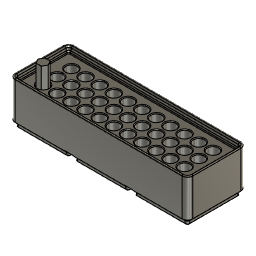
Bit holder v4 (Autodesk Fusion 360 design; units mm, degrees)
Autodesk Fusion 360 part; units mm, degrees
note: some values were not read from the file. Set by a fixed rule: which face or edge a step refers to.
sketch "Sketch1" plane through (0, 0, 0) normal (0, 0, 1) x (1, 0, 0) in component "Standard Bit"
  line L0 (-1.8331, 3.175) -> (-3.6662, 0)
  line L1 (-3.6662, 0) -> (-1.8331, -3.175)
  line L2 (-1.8331, -3.175) -> (1.8331, -3.175)
  line L3 (1.8331, -3.175) -> (3.6662, 0)
  line L4 (3.6662, 0) -> (1.8331, 3.175)
  line L5 (1.8331, 3.175) -> (-1.8331, 3.175)
  dimension "d234" = 6.35
  measures "d234" distance of L2 L5
extrude "Extrude2" add sketch "Sketch1" along normal blind 8 makes body 1 in component "Standard Bit"
chamfer "Chamfer1" distance 1 angle 45 6 edges at (-2.7496, -1.5875, 0) (0, -3.175, 0) (2.7496, -1.5875, 0) (2.7496, 1.5875, 0) (0, 3.175, 0) (-2.7496, 1.5875, 0) on bodies 1 in component "Standard Bit"
sketch "Sketch2" plane through (0, 0, 8) normal (0, 0, 1) x (-1, 0, 0) in component "Standard Bit"
  line L0 (-1.8331, -3.175) -> (1.8331, -3.175)
  line L1 (1.8331, -3.175) -> (3.6662, 0)
  line L2 (3.6662, 0) -> (1.8331, 3.175)
  line L3 (1.8331, 3.175) -> (-1.8331, 3.175)
  line L4 (-1.8331, 3.175) -> (-3.6662, 0)
  line L5 (-3.6662, 0) -> (-1.8331, -3.175)
  circle A0 centre (0, 0) radius 3.6662
  constraint coincident A0.centre origin
  constraint coincident L0.start A0
extrude "Extrude1" add sketch "Sketch1" along normal blind 17 from surface at 8 bodies 1 in component "Standard Bit"
pipe "Pipe1" cut square section size 0.5 path "Sketch2" along A0 bodies 1 in component "Standard Bit"
sketch "Sketch1 (2)" plane through (0, 0, 0) normal (0, 0, 1) x (1, 0, 0) in component "Blank Storage"
  line L0 (0, 42) -> (42, 42)
  line L1 (42, 42) -> (42, 0)
  line L2 (42, 0) -> (0, 0)
  line L3 (0, 0) -> (0, 42)
  line L4 (0, 42) -> (42, 0) construction
  line L5 (42, 21) -> (0, 21) construction
  line L6 (42, 14.5) -> (0, 14.5)
  line L7 (42, 27.5) -> (0, 27.5)
  line L8 (27.5, 42) -> (27.5, 0)
  line L9 (14.5, 42) -> (14.5, 0)
  line L10 (14.5, 14.5) -> (0, 0) construction
  circle A0 centre (8, 8) radius 1.5
  circle A1 centre (34, 8) radius 1.5
  circle A2 centre (34, 34) radius 1.5
  circle A3 centre (8, 34) radius 1.5
  circle A4 centre (8, 8) radius 3.25
  circle A5 centre (34, 8) radius 3.25
  circle A6 centre (34, 34) radius 3.25
  circle A7 centre (8, 34) radius 3.25
  line L11 (6.5, 10.8831) -> (6.5, 5.1169)
  line L12 (5.1169, 6.5) -> (10.8831, 6.5)
  line L13 (9.5, 5.1169) -> (9.5, 10.8831)
  line L14 (10.8831, 9.5) -> (5.1169, 9.5)
  point P0 (21, 21)
  dimension "d1" = 42
  dimension "d2" = 42
  dimension "d65" = 13
  dimension "d67" = 90
  dimension "d69" = 3
  dimension "d71" = 360
  dimension "d80" = 6.5
  dimension "d85" = 8
  constraint horizontal L0
  constraint perpendicular L0 L1
  constraint parallel L0 L2
  constraint parallel L1 L3
  constraint coincident L2.end L3.start
  constraint midpoint L1 L5.start
  constraint midpoint L3 L5.end
  constraint coincident L1 L6.start
  constraint coincident L3 L6.end
  constraint perpendicular L3 L6
  constraint symmetric L5 L6.start L7.start
  constraint symmetric L5 L6.end L7.end
  constraint midpoint L4 P0
  constraint coincident L9 L10.start
  constraint coincident L6 L10.start
  constraint concentric A0 A4
  constraint coincident L10 A0.centre
  constraint coincident A4 L11.start
  constraint coincident A4 L11.end
  constraint coincident A4 L12.start
  constraint coincident A4 L12.end
  constraint coincident A4 L13.start
  constraint coincident A4 L13.end
  constraint coincident A4 L14.start
  constraint coincident A4 L14.end
  constraint horizontal L12
  constraint horizontal L14
  constraint vertical L13
  constraint vertical L11
  constraint tangent A0 L11
  constraint tangent A0 L12
  constraint tangent A0 L13
  constraint tangent A0 L14
  measures "d1" distance of L1.end L2.end
  measures "d2" distance of L0.end L1.end
  measures "d65" distance of L6 L7
  measures "d69" diameter of A0
  measures "d80" diameter of A4
  measures "d85" distance of L2 A0.centre
extrude "Extrude1'" add sketch "Sketch1 (2)" along normal blind 5 separate body contours L0 L3 L7 L9 | L0 L7 L8 L9 | L3 L6 L7 L9 | L0 L1 L7 L8 | L6 L7 L8 L9 | L2 L3 L6 L9 | L1 L6 L7 L8 | L2 L6 L8 L9 | L1 L2 L6 L8 | A0 | A0 L12 L13 | A4 L12 L13 L14 | A0 L13 L14 | A4 L11 L13 L14 | A0 L11 L14 | A0 L11 L12 | A4 L11 L12 L13 | A4 L12 L13 | A4 L13 L14 | A4 L11 L12 L14 | A4 L11 L14 | A4 L11 L12 | A1 | A2 | A3 | A5 | A6 | A7 makes body 2 in component "Blank Storage"
ref_plane "WorkPlane1" through (21, 21, 2.5) normal (0, -1, 0) x (1, 0, 0) in component "Blank Storage"
sketch "Sketch2 (2)" plane through (0, 21, 0) normal (0, -1, 0) x (1, 0, 0) in component "Blank Storage"
  line L0 (42, 0) -> (0, 0)
  line L1 (0, 0) -> (0, 5)
  line L2 (3.2, 0) -> (2.4, 0.8)
  line L3 (3.2, 0) -> (0, 0) construction
  line L4 (2.4, 0.8) -> (2.4, 2.6)
  line L5 (2.4, 2.6) -> (0, 5)
  line L6 (0, 5) -> (-5.1222, 5)
  line L7 (-5.1222, 5) -> (-5.1222, -0.0937)
  line L8 (-5.1222, -0.0937) -> (0, 0)
  dimension "d39" = 45
  dimension "d40" = 45
  dimension "d41" = 0.8
  dimension "d43" = 5
  dimension "d112" = 2.4
  constraint horizontal L3
  constraint coincident L0 L2.start
  constraint perpendicular L0 L4
  constraint coincident L1 L5.end
  constraint coincident L0.end L1.start
  constraint coincident L1.end L5.end
  constraint perpendicular L1 L6
  constraint perpendicular L6 L7
  measures "d39" angle of L2 L3
  measures "d40" angle of L4 L5
  measures "d41" distance of L2.end L3
  measures "d43" distance of L3 L1.end
  measures "d112" horizontal distance of L0.end L2.end
sketch "Sketch3" plane through (0, 0, 0) normal (0, 0, -1) x (1, 0, 0) in component "Storage Template v5"
  line L0 (42, 0) -> (0, 0)
  line L1 (0, 0) -> (0, -42)
  line L2 (0, -42) -> (42, -42)
  line L3 (42, -42) -> (42, 0)
  arc A0 (4, 0) -> (0, -4) centre (4, -4) ccw
  line L4 (0, -42) -> (42, 0) construction
  arc A1 (0, -38) -> (4, -42) centre (4, -38) ccw
  arc A2 (38, -42) -> (42, -38) centre (38, -38) ccw
  arc A3 (42, -4) -> (38, 0) centre (38, -4) ccw
  line L5 (0, -4) -> (0, -38)
  line L6 (4, -42) -> (38, -42)
  line L7 (42, -38) -> (42, -4)
  line L8 (38, 0) -> (4, 0)
  point P0 (21, -21)
  dimension "d37" = 360
  constraint coincident L1.end L2.start
  constraint coincident L0.start L3.end
  constraint midpoint L4 P0
sweep "Sweep1" cut profiles "Sketch2 (2)" path "Sketch3" along L8 A0 L5 A1 L6 A2 L7 A3 section 1 bodies 2 in component "Blank Storage"
extrude "Extrude3" [suppressed] in component "Blank Storage"
draft "Draft1" [suppressed] in component "Blank Storage"
extrude "Extrude4" cut sketch "Sketch1 (2)" along normal up to surface (5 mm away) contours A0 | A1 | A2 | A3 bodies 2 in component "Blank Storage"
extrude "Extrude5" cut sketch "Sketch1 (2)" along normal blind 2.4 contours A0 L12 L13 | A4 L12 L13 L14 | A0 L13 L14 | A4 L11 L13 L14 | A0 L11 L14 | A0 L11 L12 | A4 L11 L12 L13 | A4 L12 L13 | A4 L13 L14 | A4 L11 L12 L14 | A4 L11 L14 | A4 L11 L12 | A5 | A6 | A7 bodies 2 in component "Blank Storage"
extrude "Extrude8" cut sketch "Sketch1 (2)" along normal blind 0.25 from surface at 2.4 contours A0 L12 L13 | A4 L12 L13 L14 | A0 L13 L14 | A0 L11 L14 | A0 L11 L12 | A4 L11 L12 L14 bodies 2 in component "Blank Storage"
extrude "Extrude9" cut sketch "Sketch1 (2)" along normal blind 0.25 from surface at 2.65 contours A0 L12 L13 | A0 L13 L14 | A4 L11 L13 L14 | A0 L11 L14 | A0 L11 L12 | A4 L11 L12 L13 bodies 2 in component "Blank Storage"
pattern_circular "C-Pattern1" count 4 over 360 about axis through (21, 21, -42) along (0, 0, 1) of "Extrude8", "Extrude9" in component "Blank Storage"
pattern_linear "R-Pattern1" count 3 spacing 42 along (1, 0, 0) of bodies 2 makes body 3 at (66.9668, 17.0068, 5) makes body 4 at (108.9668, 17.0068, 5) in component "Blank Storage"
sketch "Sketch4" plane through (0, 0, 5) normal (0, 0, 1) x (-1, 0, 0) in component "Blank Storage"
  line L0 (-4, 0) -> (-122, 0)
  line L1 (-126, -4) -> (-126, -38)
  line L2 (-122, -42) -> (-4, -42)
  line L3 (0, -38) -> (0, -4)
  arc A0 (0, -4) -> (-4, 0) centre (-4, -4) ccw
  arc A1 (-122, 0) -> (-126, -4) centre (-122, -4) ccw
  arc A2 (-126, -38) -> (-122, -42) centre (-122, -38) ccw
  arc A3 (-4, -42) -> (0, -38) centre (-4, -38) ccw
  line L4 (-122, -41.75) -> (-4, -41.75)
  arc A4 (-4, -41.75) -> (-0.25, -38) centre (-4, -38) ccw
  line L5 (-0.25, -38) -> (-0.25, -4)
  arc A5 (-0.25, -4) -> (-4, -0.25) centre (-4, -4) ccw
  line L6 (-4, -0.25) -> (-122, -0.25)
  arc A6 (-122, -0.25) -> (-125.75, -4) centre (-122, -4) ccw
  line L7 (-125.75, -4) -> (-125.75, -38)
  arc A7 (-125.75, -38) -> (-122, -41.75) centre (-122, -38) ccw
  point P0 (-126, 0)
  point P1 (0, -42)
  dimension "d44" = 126
  dimension "d45" = 42
  dimension "d48" = 4
  dimension "d49" = 4
  dimension "d50" = 4
  dimension "d51" = 4
  dimension "d118" = -0.25
  constraint horizontal L0
  constraint vertical L1
  constraint horizontal L2
  constraint vertical L3
  constraint coincident origin L0
  constraint coincident origin L3
  constraint tangent L0 A0
  constraint tangent L3 A0
  constraint coincident P0 L0
  constraint coincident P0 L1
  constraint tangent L0 A1
  constraint tangent L1 A1
  constraint tangent L1 A2
  constraint tangent L2 A2
  constraint coincident P1 L2
  constraint coincident P1 L3
  constraint tangent L2 A3
  constraint tangent L3 A3
  measures "d44" distance of origin P0
  measures "d45" distance of origin P1
  measures "d48" radius of A0
  measures "d49" radius of A1
  measures "d50" radius of A2
  measures "d51" radius of A3
extrude "Extrude2'" add sketch "Sketch4" along normal blind 23 contours L0 L1 L2 L3 A0 A1 A2 A3 | L4 A4 L5 A5 L6 A6 L7 A7 bodies 2 3 4 in component "Blank Storage"
sketch "Sketch5" plane through (21, 21, 2.5) normal (0, -1, 0) x (1, 0, 0) in component "Blank Storage"
  line L0 (-18.6, 0.1) -> (-21, 2.5)
  line L1 (101, 2.5) -> (-17, 2.5)
  line L2 (-18.6, -1.7) -> (-18.6, 0.1)
  line L3 (-17.8, -2.5) -> (-18.6, -1.7)
  line L4 (-17, 25.5) -> (-21, 25.5)
  line L5 (-17, 25.5) -> (-21, 25.5)
  line L6 (-17, 25.5) -> (101, 25.5)
  line L7 (105, 25.5) -> (101, 25.5)
  line L8 (105, 25.5) -> (101, 25.5)
  line L9 (101, 25.5) -> (-17, 25.5)
  line L10 (-18.6, 28.1) -> (-21, 30.5)
  line L11 (-18.6, 26.3) -> (-18.6, 28.1)
  line L12 (-17.8, 25.5) -> (-18.6, 26.3)
  line L13 (-21, 2.5) -> (-21, 25.5)
  line L14 (-21, 25.5) -> (-21, 2.5)
  line L15 (-17.8, 25.5) -> (-21, 25.5)
  line L16 (-21, 30.5) -> (-21, 25.5)
  line L17 (-17.9768, 25.3232) -> (-18.85, 26.1964)
  line L18 (-18.85, 26.1964) -> (-18.85, 27.9964)
  line L19 (-18.85, 27.9964) -> (-21.1768, 30.3232)
  dimension "d54" = 0
  dimension "d55" = 28
  dimension "d56" = -0.25
  constraint coincident L14 L4.end
  constraint perpendicular L14 L15
sweep "Sweep2" add profiles "Sketch5" along 8 edges at (63, 0, 28) (124.8284, 1.1716, 28) (126, 21, 28) (124.8284, 40.8284, 28) (63, 42, 28) (1.1716, 40.8284, 28) (0, 21, 28) (1.1716, 1.1716, 28) section 1 contours L4 L5 L15 L16 L17 L18 L19 on bodies 2 bodies 2 in component "Blank Storage"
extrude "Extrude2''" cut sketch "Sketch4" along normal through all and the other way through all bodies 2 in component "Blank Storage"
fillet "Fillet2" radius 0.6 8 edges at (63, 0.25, 32.3964) (124.6517, 1.3483, 32.3964) (125.75, 21, 32.3964) (124.6517, 40.6517, 32.3964) (63, 41.75, 32.3964) (1.3483, 40.6517, 32.3964) (0.25, 21, 32.3964) (1.3483, 1.3483, 32.3964) on bodies 2 in component "Blank Storage"
extrude "Extrude1''" cut 1 faces at (43.3333, 27.0512, 28) along direction (0, 0, -1) blind 1 on bodies 2 bodies 2 in component "Blank Storage"
sketch "Sketch7" plane through (0, 0, 27) normal (0, 0, 1) x (-1, 0, 0)
  line L0 (-0.25, -4) -> (-0.25, -38)
  line L1 (-4, -41.75) -> (-80, -41.75)
  line L2 (-3.25, -30.8529) -> (-13.1471, -30.8529) construction
  line L3 (-13.1471, -30.8529) -> (-13.1471, -40.75) construction
  line L4 (-11.1986, -34.2279) -> (-9.25, -30.8529)
  line L5 (-9.25, -30.8529) -> (-11.1986, -27.4779)
  line L6 (-11.1986, -27.4779) -> (-15.0957, -27.4779)
  line L7 (-15.0957, -27.4779) -> (-17.0442, -30.8529)
  line L8 (-17.0442, -30.8529) -> (-15.0957, -34.2279)
  line L9 (-15.0957, -34.2279) -> (-11.1986, -34.2279)
  circle A0 centre (-13.1471, -30.8529) radius 3.8971
  line L10 (-0.25, -38) -> (-0.25, -4)
  line L11 (-80, -41.75) -> (-4, -41.75)
  arc A1 (-4, -39.1536) -> (-2.8464, -38) centre (-4, -38) ccw
  line L12 (-2.8464, -38) -> (-2.8464, -4)
  arc A2 (-2.8464, -4) -> (-4, -2.8464) centre (-4, -4) ccw
  line L13 (-4, -2.8464) -> (-122, -2.8464)
  arc A3 (-122, -2.8464) -> (-123.1536, -4) centre (-122, -4) ccw
  line L14 (-123.1536, -4) -> (-123.1536, -38)
  arc A4 (-123.1536, -38) -> (-122, -39.1536) centre (-122, -38) ccw
  line L15 (-122, -39.1536) -> (-4, -39.1536)
  line L16 (-0.25, -38) -> (-0.25, -4)
  point P0 (-13.1471, -30.8529)
  point P1 (-13.1471, -34.75)
  point P2 (-9.25, -30.8529)
  dimension "d302" = 6.75
  dimension "d305" = 7
  dimension "d327" = 9
  constraint coincident P0 L2.end
  constraint coincident P2 A0
  constraint coincident A0 P1
  constraint coincident A0 P2
  constraint coincident L2 P2
  constraint coincident L3 P1
  constraint horizontal L9
  measures "d302" distance of L6 L9
  measures "d305" distance of L1 P1
  measures "d327" distance of P2 L16
extrude "Extrude10" cut sketch "Sketch7" against normal blind 6 contours L4 L5 L6 L7 L8 L9 | L9 A0 | L4 A0 | L5 A0 | L8 A0 | L6 A0 | L7 A0 bodies 2 in component "Blank Storage"
extrude "Extrude11" cut sketch "Sketch7" against normal blind 11 contours L4 L5 L6 L7 L8 L9 bodies 2 in component "Blank Storage"
fillet "Fillet7" radius 0.5 1 edges at (16.7805, 29.4436, 27) on bodies 2 in component "Blank Storage"
pattern_linear "R-Pattern2" count 3 spacing 10 along (0, -1, 0) count 11 spacing 10 along (1, 0, 0) of "Extrude10", "Extrude11", "Fillet7" in component "Blank Storage"
component "Standard Bit" placed x (1, 0, 0) y (0, 1, 0) z (0, 0, 1) at (13.1471, 10.8529, 16)
component "Storage Template v5" placed x (1, 0, 0) y (0, 1, 0) z (0, 0, 1) at (0, 0, 0)
component "Blank Storage" placed x (1, 0, 0) y (0, 1, 0) z (0, 0, 1) at (0, 0, 0) in component "Storage Template v5"
equation "slotsWide = 2"
equation "slotsHigh = 2 / 3"
equation "slotsDeep = 1"
equation "slotDimension = 42 mm"
equation "nestingDepth = 5 mm"
equation "nestingRimWidth = 2.4 mm"
equation "nestingClearance = 0.25 mm"
equation "cornerFillet = 4 mm"
equation "ledStripWidth = 13 mm"
equation "ledSlotHeight = 4 mm"
equation "screwTightDiameter = 3 mm"
equation "magnetDiameter = 6.5 mm"
equation "magnetThiccness = 2.4 mm"
equation "wallThiccness = 1.2 mm"
equation "d234 = BitDiameter"
equation "d235 = 25 mm - 8 mm"
equation "BitDiameter = 6.35 mm" comment "1/4 Zoll"
equation "BitsW = 3"
equation "BitsH = 11"
equation "d302 = BitDiameter + 0.4 mm"
equation "d1 = slotDimension"
equation "d2 = slotDimension"
equation "d3 = nestingDepth"
equation "slotsWide_1 = 3"
equation "slotsHigh_1 = 2 / 3"
equation "slotsDeep_1 = 1"
equation "slotDimension_1 = 42 mm"
equation "nestingDepth_1 = 5 mm"
equation "nestingRimWidth_1 = 2.4 mm"
equation "nestingClearance_1 = 0.25 mm"
equation "cornerFillet_1 = 4 mm"
equation "d31 = slotsWide_1"
equation "d32 = slotsDeep_1"
equation "d33 = slotDimension_1"
equation "d34 = slotDimension_1"
equation "d38 = -slotDimension_1 / 2"
equation "d43 = nestingDepth_1"
equation "d44 = slotDimension_1 * slotsWide_1"
equation "d45 = slotDimension_1 * slotsDeep_1"
equation "d46 = slotDimension_1 * slotsHigh_1 - nestingDepth_1"
equation "d48 = cornerFillet_1"
equation "d49 = cornerFillet_1"
equation "d50 = cornerFillet_1"
equation "d51 = cornerFillet_1"
equation "d55 = slotDimension_1 * slotsHigh_1"
equation "d56 = -nestingClearance_1"
equation "ledStripWidth_1 = 13 mm"
equation "ledSlotHeight_1 = 4 mm"
equation "d65 = ledStripWidth_1"
equation "screwTightDiameter_1 = 3 mm"
equation "d69 = screwTightDiameter_1"
equation "d72 = ledSlotHeight_1"
equation "magnetDiameter_1 = 6.5 mm"
equation "magnetThiccness_1 = 2.4 mm"
equation "d80 = magnetDiameter_1"
equation "d81 = magnetThiccness_1"
equation "wallThiccness_1 = 1.2 mm"
equation "d112 = nestingRimWidth_1"
equation "d122 = -resess"
equation "d211_1 = 360.0 deg"
equation "d225 = layerHeight"
equation "d228 = layerHeight"
equation "layerHeight = 0.25 mm"
equation "resess = 1 mm"
equation "d319 = BitsW"
equation "d320 = BitsH"
